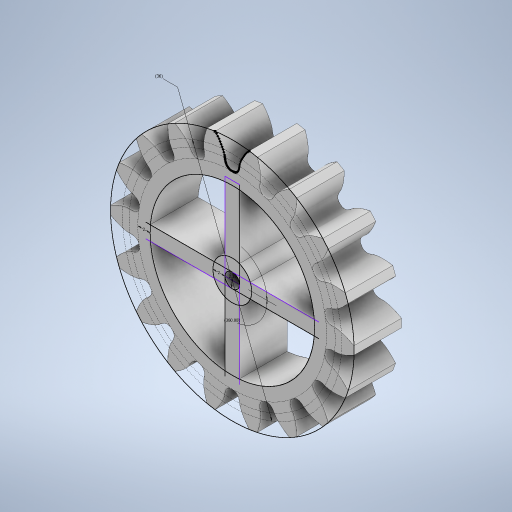
# Autodesk Inventor part: gear_V2
Saved by Autodesk Inventor 2023 (Build 270158000, 158)
## iProperties
Created: 2022-11-22
Part Number: gear_V2
Material: Generic
Document SubType Name: Modeling
Designer: shrey
Density: 1 g/cm^3
Appearance: Default
Author: shrey
Autodesk Inventor part; units mm, degrees
ref_plane "YZ Plane" through (0, 0, 0) normal (1, 0, 0) x (0, 1, 0)
ref_plane "XZ Plane" through (0, 0, 0) normal (0, 1, 0) x (-1, 0, 0)
ref_plane "XY Plane" through (0, 0, 0) normal (0, 0, 1) x (1, 0, 0)
sketch "Sketch1" plane through (0, 0, 0) normal (0, 0, 1) x (1, 0, 0)
  spline S0 degree 3 poles (-2.7997, 19.8031) (-2.7271, 19.7161) (-2.5819, 19.542) (-2.3756, 19.2717) (-2.1785, 18.9948) (-1.9921, 18.7104) (-1.8177, 18.4185) (-1.6565, 18.1191) (-1.5108, 17.8119) (-1.3828, 17.4967) (-1.2964, 17.2268) (-1.241, 17.0068) (-1.2198, 16.838) (-1.2001, 16.6693) (-1.1697, 16.5018) (-1.1239, 16.338) (-1.0671, 16.1777) (-0.9919, 16.0248) (-0.8982, 15.8826) (-0.7854, 15.7546) (-0.6735, 15.6669) (-0.5777, 15.6062) (-0.5004, 15.5705) (-0.4213, 15.5391) (-0.3387, 15.5188) (-0.255, 15.5031) (-0.1416, 15.4981) (0, 15.5013) (0.1416, 15.4981) (0.255, 15.5031) (0.3387, 15.5188) (0.4213, 15.5391) (0.5004, 15.5705) (0.5777, 15.6062) (0.6735, 15.6669) (0.7854, 15.7546) (0.8982, 15.8826) (0.9919, 16.0248) (1.0671, 16.1777) (1.1239, 16.338) (1.1697, 16.5018) (1.2001, 16.6693) (1.2198, 16.838) (1.241, 17.0068) (1.2964, 17.2268) (1.3828, 17.4967) (1.5108, 17.8119) (1.6565, 18.1191) (1.8177, 18.4185) (1.9921, 18.7104) (2.1785, 18.9948) (2.3756, 19.2717) (2.5819, 19.542) (2.7271, 19.7161) (2.7997, 19.8031) knots 0 0 0 0 0.033991 0.067983 0.101975 0.135966 0.169957 0.203948 0.237937 0.271925 0.305908 0.322902 0.339886 0.356881 0.373875 0.390866 0.407855 0.424845 0.441833 0.458817 0.47579 0.484288 0.492785 0.501283 0.509779 0.518277 0.526773 0.543769 0.560766 0.569261 0.577759 0.586255 0.594754 0.60325 0.611748 0.628722 0.645705 0.662693 0.679683 0.696672 0.713663 0.730657 0.747652 0.764636 0.78163 0.815614 0.849601 0.883591 0.917581 0.951572 0.985563 1.019555 1.053547 1.087538 1.087538 1.087538 1.087538
  circle A0 centre (0, 0) radius 15.5 construction
  circle A1 centre (0, 0) radius 16.9145 construction
  circle A2 centre (0, 0) radius 18 construction
  circle A3 centre (0, 0) radius 20
  point P0 (-2.5838, 19.5405)
  point P1 (-2.3771, 19.2706)
  point P2 (-2.1803, 18.9935)
  point P3 (-1.9941, 18.7091)
  point P4 (-1.8199, 18.4173)
  point P5 (-1.6591, 18.1178)
  point P6 (-1.5137, 17.8105)
  point P7 (-1.3869, 17.4952)
  point P8 (-1.2837, 17.1715)
  point P9 (-1.2444, 17.0061)
  point P10 (-1.2201, 16.838)
  point P11 (-1.1984, 16.6695)
  point P12 (-1.1671, 16.5024)
  point P13 (-1.1221, 16.3386)
  point P14 (-1.0641, 16.1789)
  point P15 (-0.9888, 16.0266)
  point P16 (-0.895, 15.8849)
  point P17 (-0.7818, 15.7583)
  point P18 (-0.6491, 15.6526)
  point P19 (-0.5768, 15.6079)
  point P20 (-0.5001, 15.5712)
  point P21 (-0.4207, 15.541)
  point P22 (-0.3385, 15.5195)
  point P23 (-0.2548, 15.5051)
  point P24 (-0.17, 15.5)
  point P25 (0, 15.5)
  point P26 (0.17, 15.5)
  point P27 (0.2548, 15.5051)
  point P28 (0.3385, 15.5195)
  point P29 (0.4207, 15.541)
  point P30 (0.5001, 15.5712)
  point P31 (0.5768, 15.6079)
  point P32 (0.6491, 15.6526)
  point P33 (0.7818, 15.7583)
  point P34 (0.895, 15.8849)
  point P35 (0.9888, 16.0266)
  point P36 (1.0641, 16.1789)
  point P37 (1.1221, 16.3386)
  point P38 (1.1671, 16.5024)
  point P39 (1.1984, 16.6695)
  point P40 (1.2201, 16.838)
  point P41 (1.2444, 17.0061)
  point P42 (1.2837, 17.1715)
  point P43 (1.3869, 17.4952)
  point P44 (1.5137, 17.8105)
  point P45 (1.6591, 18.1178)
  point P46 (1.8199, 18.4173)
  point P47 (1.9941, 18.7091)
  point P48 (2.1803, 18.9935)
  point P49 (2.3771, 19.2706)
  point P50 (2.5838, 19.5405)
  dimension "d10" = 36
  constraints: 4 centre point, 2 point on circle, 111 other
  measures "d10" diameter of A2
extrude "Extrusion1" add sketch "Sketch1" against normal blind 7.82
extrude "Extrusion2" cut sketch "Sketch1" against normal through all contours A3 S0 picked at (-0.2701, 18.4272)
pattern_circular "Circular Pattern1" count 18 over 360 about axis through (0, 0, 0) along (0, 0, -1) of "Extrusion2"
sketch "Sketch2" plane through (0, 0, 0) normal (0, 0, 1) x (1, 0, 0)
  circle A0 centre (0, 0) radius 1.185
  circle A1 centre (0, 0) radius 3.185
  circle A2 centre (0, 0) radius 15.5 construction
  circle A3 centre (0, 0) radius 13.5
  line L0 (-1.185, 0) -> (1.185, 0)
  line L1 (1.185, 0) -> (1.185, 14.215)
  line L2 (1.185, 14.215) -> (-1.185, 14.215)
  line L3 (-1.185, 14.215) -> (-1.185, 0)
  line L4 (0, 1.185) -> (-14.215, 1.185)
  line L5 (-14.215, -1.185) -> (0, -1.185)
  line L6 (-1.185, 0) -> (-1.185, -14.215)
  line L7 (1.185, -14.215) -> (1.185, 0)
  line L8 (0, -1.185) -> (14.215, -1.185)
  line L9 (14.215, 1.185) -> (0, 1.185)
  point P0 (-1.185, -13.4479)
  point P1 (-1.185, -2.9563)
  point P2 (-2.9563, -1.185)
  point P3 (-13.4479, -1.185)
  point P4 (13.4479, -1.185)
  point P5 (2.9563, -1.185)
  point P6 (1.185, -2.9563)
  point P7 (1.185, -13.4479)
  point P8 (2.9563, 1.185)
  point P9 (13.4479, 1.185)
  point P10 (1.185, 13.4479)
  point P11 (1.185, 2.9563)
  point P12 (-13.4479, 1.185)
  point P13 (-2.9563, 1.185)
  point P14 (-1.185, 2.9563)
  point P15 (-1.185, 13.4479)
  dimension "d7" = 2.37
  dimension "d11" = 2
  dimension "d12" = 2
  dimension "d15" = 360
  constraints: 20 end point, 2 centre point, 2 parallel, 1 coincident, 1 horizontal, 1 horizontal alignment, 1 perpendicular, 1 vertical, 27 other
  measures "d12" radial gap between concentric circles of A2 A3
extrude "Extrusion3" cut sketch "Sketch2" against normal through all contours L0 A0 | A0 L0 | L1 A3 L9 A1 | A1 L8 A3 L7 | A1 L4 A3 L3 | A1 L6 A3 L5
equation "\"Module\" = 2"
equation "\"PressureAngle\" = 20deg"
equation "\"UnitProfileClearance\" = 0.25"
equation "\"UnitRoundRadius\" = 0.35"
equation "\"RootDiameter\" = 31"
equation "\"BaseDiameter\" = 33.82893"
equation "\"PitchDiameter\" = 36"
equation "\"HelixAngle\" = 0"
equation "\"UnitCorrection\" = 0"
equation "\"UnitAddendumModification\" = 0"
equation "\"CircularPitch\" = 6.283185"
equation "\"UnitBacklashShift\" = 0"
equation "\"TotalToolShift\" = 0"
equation "\"IsInternal\" = 0"
body "Solid1"
